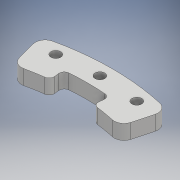
# Autodesk Inventor part: bump_sensor_mount
Saved by Autodesk Inventor 2017.2 (Build 212233000, 233)
## iProperties
Created: 2017-10-26
Part Number: bump_sensor_mount
Material: Generic
Document SubType Name: Modeling
Designer: Nic
Density: 1 g/cm^3
Appearance: Default
Author: Nic
Autodesk Inventor part; units mm, degrees
ref_plane "YZ Plane" through (0, 0, 0) normal (1, 0, 0) x (0, 1, 0)
ref_plane "XZ Plane" through (0, 0, 0) normal (0, 1, 0) x (-1, 0, 0)
ref_plane "XY Plane" through (0, 0, 0) normal (0, 0, 1) x (1, 0, 0)
sketch "Sketch1" plane through (0, 0, 0) normal (0, 0, 1) x (1, 0, 0)
  circle A0 centre (0, 0) radius 1
  arc A1 (10.9174, 1.2936) -> (-10.9174, 1.2936) centre (0, -47.5) ccw
  line L0 (-11.3763, -5.0432) -> (-12.4125, -1.1758)
  line L1 (0, -47.5) -> (0, 2.5) construction
  line L2 (11.3763, -5.0432) -> (12.4125, -1.1758)
  line L3 (-10.8704, -6.9311) -> (0, -47.5) construction
  line L4 (-4.4935, -4.7471) -> (-4.5981, -3.7523)
  line L5 (4.4935, -4.7471) -> (4.5981, -3.7523)
  arc A2 (9.0151, -6.4789) -> (5.3604, -5.8435) centre (0, -47.5) ccw
  arc A3 (-5.3604, -5.8435) -> (-9.0151, -6.4789) centre (0, -47.5) ccw
  line L6 (0, -47.5) -> (-4.3902, -5.7301) construction
  arc A4 (3.6854, -2.6512) -> (-3.6854, -2.6512) centre (0, -47.5) ccw
  circle A5 centre (0, -47.5) radius 47.5 construction
  circle A6 centre (8.2483, -0.7216) radius 1
  circle A7 centre (-8.2483, -0.7216) radius 1
  line L7 (0, -47.5) -> (-8.2483, -0.7216) construction
  arc A8 (-10.9174, 1.2936) -> (-12.4125, -1.1758) centre (-10.4807, -0.6582) ccw
  arc A9 (-11.3763, -5.0432) -> (-9.0151, -6.4789) centre (-9.4444, -4.5256) ccw
  arc A10 (12.4125, -1.1758) -> (10.9174, 1.2936) centre (10.4807, -0.6582) ccw
  arc A11 (9.0151, -6.4789) -> (11.3763, -5.0432) centre (9.4444, -4.5256) ccw
  arc A12 (-3.6854, -2.6512) -> (-4.5981, -3.7523) centre (-3.6035, -3.6478) ccw
  arc A13 (4.5981, -3.7523) -> (3.6854, -2.6512) centre (3.6035, -3.6478) ccw
  arc A14 (4.4935, -4.7471) -> (5.3604, -5.8435) centre (5.488, -4.8517) ccw
  arc A15 (-5.3604, -5.8435) -> (-4.4935, -4.7471) centre (-5.488, -4.8517) ccw
  point P0 (-12.941, 0.7963)
  point P1 (12.941, 0.7963)
  point P2 (-10.8704, -6.9311)
  point P3 (10.8704, -6.9311)
  point P4 (-4.7038, -2.7465)
  point P5 (4.7038, -2.7465)
  point P6 (-4.3902, -5.7301)
  point P7 (4.3902, -5.7301)
  dimension "d0" = 2
  dimension "d1" = 100
  dimension "d2" = 47.5
  dimension "d4" = 30
  dimension "d5" = 15
  dimension "d7" = 12
  dimension "d8" = 42
  dimension "d9" = 45
  dimension "d10" = 2
  dimension "d11" = 10
  dimension "d12" = 2
  dimension "d13" = 1
  constraints: 36 point on circle, 16 centre point, 16 end point, 16 tangent, 8 point on line, 7 equal radius, 4 coincident, 3 symmetric about line, 2 collinear, 1 vertical, 1 vertical alignment, 2 other
  measures "d0" diameter of A0
  measures "d1" diameter of A1
  measures "d2" distance of point (0, 0) A1.centre
  measures "d4" angle of L2 L0
  measures "d5" angle of L1 L3
  measures "d7" angle of L5 L4
  measures "d8" radius of A2
  measures "d9" radius of A4
  measures "d10" diameter of A6
  measures "d11" angle of L1 L7
  measures "d12" radius of A8
  measures "d13" radius of A12
extrude "Extrusion1" add sketch "Sketch1" along normal blind 3
body "Solid1"
